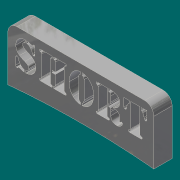
# Autodesk Inventor part: A1-19010-100-03 Tab - SHORT
Saved by Autodesk Inventor 2017 SP1 (Build 210196100, 196)
## iProperties
Created: 2014-10-23
Part Number: A1-19010-100-03 Tab - SHORT
Material: Steel, Mild
Description: 4" x 1 1/2" x 1/2" PLATE, A516 Gr.70
Document SubType Name: Modeling
Designer: Graeme_Van_Dongen
Density: 7.86 g/cm^3
Appearance: Steel
Mass: 266.205 g
Surface Area: 155.61 cm^2
Volume: 33.8683 cm^3
Author: Graeme_Van_Dongen
Autodesk Inventor part; units mm, degrees
ref_plane "YZ Plane" through (0, 0, 0) normal (1, 0, 0) x (0, 1, 0)
ref_plane "XZ Plane" through (0, 0, 0) normal (0, 1, 0) x (-1, 0, 0)
ref_plane "XY Plane" through (0, 0, 0) normal (0, 0, 1) x (1, 0, 0)
sketch "Sketch1" plane through (0, 0, 0) normal (0, 0, 1) x (1, 0, 0)
  arc A0 (50.8, 543.7321) -> (-50.8, 543.7321) centre (0, 0) ccw
  line L0 (50.8, 543.7321) -> (50.8, 581.8321)
  line L1 (50.8, 581.8321) -> (-50.8, 581.8321)
  line L2 (-50.8, 581.8321) -> (-50.8, 543.7321)
  point P0 (0, 581.8321)
  dimension "d0" = 101.6
  dimension "d1" = 38.1
  dimension "d2" = 546.1
  constraints: 6 end point, 2 parallel, 2 point on circle, 1 centre point, 1 coincident, 1 midpoint, 1 perpendicular, 1 vertical, 1 vertical alignment
  measures "d0" distance of L0.end L1.end
  measures "d1" distance of L0.start L0.end
  measures "d2" radius of A0
extrude "Extrusion1" add sketch "Sketch1" along normal mid plane 12.7
sketch "Sketch2" plane through (0, 0, 6.35) normal (0, 0, 1) x (1, 0, 0)
  line L0 (-46.29, 576.8125) -> (46.3638, 576.8125) construction
  line L1 (46.3638, 576.8125) -> (46.3638, 557.0018) construction
  line L2 (46.3638, 557.0018) -> (-46.29, 557.0018) construction
  line L3 (-46.29, 557.0018) -> (-46.29, 576.8125) construction
  line L4 (-38.7163, 576.8125) -> (-38.7163, 575.2084)
  spline S0 degree 2 poles (-38.7163, 575.2084) (-39.5762, 574.9604) (-40.4857, 573.9682) (-40.4857, 573.2571) knots 0 0 0 1 2 2 2
  spline S1 degree 2 poles (-40.4857, 573.2571) (-40.4857, 572.546) (-39.725, 571.5042) (-38.8816, 571.0247) knots 0 0 0 1 2 2 2
  spline S2 degree 2 poles (-38.8816, 571.0247) (-38.3029, 570.7105) (-36.2358, 569.801) knots 0 0 0 1 1 1
  spline S3 degree 2 poles (-36.2358, 569.801) (-34.979, 569.2553) (-33.6065, 568.3789) (-32.9781, 567.7174) knots 0 0 0 1 2 2 2
  spline S4 degree 2 poles (-32.9781, 567.7174) (-31.341, 565.9976) (-31.341, 563.5998) knots 0 0 0 1 1 1
  spline S5 degree 2 poles (-31.341, 563.5998) (-31.341, 561.8139) (-33.127, 558.8208) (-34.6814, 557.9609) knots 0 0 0 1 2 2 2
  spline S6 degree 2 poles (-34.6814, 557.9609) (-35.5247, 557.5144) (-37.5257, 557.0018) (-38.3855, 557.0018) knots 0 0 0 1 2 2 2
  line L5 (-38.3855, 557.0018) -> (-38.3855, 558.5893)
  spline S7 degree 2 poles (-38.3855, 558.5893) (-37.1784, 558.8869) (-36.1035, 559.9287) (-36.1035, 560.8217) knots 0 0 0 1 2 2 2
  spline S8 degree 2 poles (-36.1035, 560.8217) (-36.1035, 561.7643) (-36.9469, 562.4753) knots 0 0 0 1 1 1
  spline S9 degree 2 poles (-36.9469, 562.4753) (-37.4926, 562.9384) (-39.0635, 563.6164) knots 0 0 0 1 1 1
  spline S10 degree 2 poles (-39.0635, 563.6164) (-40.7668, 564.377) (-42.0401, 565.022) (-42.6354, 565.4519) knots 0 0 0 1 2 2 2
  spline S11 degree 2 poles (-42.6354, 565.4519) (-45.2482, 567.3205) (-45.2482, 570.4294) knots 0 0 0 1 1 1
  spline S12 degree 2 poles (-45.2482, 570.4294) (-45.2482, 572.0169) (-43.9418, 574.7123) (-42.7677, 575.5391) knots 0 0 0 1 2 2 2
  spline S13 degree 2 poles (-42.7677, 575.5391) (-41.1306, 576.6802) (-38.7163, 576.8125) knots 0 0 0 1 1 1
  line L6 (-39.4439, 558.5893) -> (-39.4439, 557.0018)
  spline S14 degree 2 poles (-39.4439, 557.0018) (-40.5849, 557.0018) (-41.974, 557.6467) knots 0 0 0 1 1 1
  spline S15 degree 2 poles (-41.974, 557.6467) (-42.4866, 557.8947) (-42.8835, 558.027) (-43.0654, 558.027) knots 0 0 0 1 2 2 2
  spline S16 degree 2 poles (-43.0654, 558.027) (-43.3299, 558.027) (-43.6111, 557.8451) (-43.9253, 557.4813) knots 0 0 0 1 2 2 2
  spline S17 degree 2 poles (-43.9253, 557.4813) (-44.1733, 557.1837) (-44.471, 557.1837) knots 0 0 0 1 1 1
  spline S18 degree 2 poles (-44.471, 557.1837) (-45.2482, 557.1837) (-45.2482, 558.3908) knots 0 0 0 1 1 1
  line L7 (-45.2482, 558.3908) -> (-45.2482, 563.4675)
  spline S19 degree 2 poles (-45.2482, 563.4675) (-45.2482, 563.8479) (-44.8017, 564.3936) (-44.471, 564.4101) knots 0 0 0 1 2 2 2
  spline S20 degree 2 poles (-44.471, 564.4101) (-44.1568, 564.4266) (-43.8095, 564.0463) (-43.6772, 563.5668) knots 0 0 0 1 2 2 2
  spline S21 degree 2 poles (-43.6772, 563.5668) (-43.363, 562.3761) (-42.1559, 560.276) (-41.3456, 559.5649) knots 0 0 0 1 2 2 2
  spline S22 degree 2 poles (-41.3456, 559.5649) (-40.5188, 558.8043) (-39.4439, 558.5893) knots 0 0 0 1 1 1
  line L8 (-37.6083, 575.2084) -> (-37.6083, 576.7463)
  spline S23 degree 2 poles (-37.6083, 576.7463) (-36.765, 576.6802) (-35.5413, 576.3494) (-34.4168, 575.8699) knots 0 0 0 1 2 2 2
  spline S24 degree 2 poles (-34.4168, 575.8699) (-34.1357, 575.7541) (-33.9538, 575.7541) knots 0 0 0 1 1 1
  spline S25 degree 2 poles (-33.9538, 575.7541) (-33.6892, 575.7541) (-33.5569, 575.936) knots 0 0 0 1 1 1
  line L9 (-33.5569, 575.936) -> (-33.2592, 576.3494)
  spline S26 degree 2 poles (-33.2592, 576.3494) (-33.0277, 576.6636) (-32.7135, 576.6636) knots 0 0 0 1 1 1
  spline S27 degree 2 poles (-32.7135, 576.6636) (-32.3332, 576.6636) (-31.9859, 576.1179) (-31.9859, 575.5391) knots 0 0 0 1 2 2 2
  line L10 (-31.9859, 575.5391) -> (-31.9859, 570.9255)
  spline S28 degree 2 poles (-31.9859, 570.9255) (-31.9859, 570.5121) (-32.449, 569.9994) (-32.8128, 569.9994) knots 0 0 0 1 2 2 2
  spline S29 degree 2 poles (-32.8128, 569.9994) (-33.0939, 569.9994) (-33.3254, 570.1813) knots 0 0 0 1 1 1
  spline S30 degree 2 poles (-33.3254, 570.1813) (-33.4577, 570.2971) (-33.6065, 570.6113) (-33.6727, 570.9916) knots 0 0 0 1 2 2 2
  spline S31 degree 2 poles (-33.6727, 570.9916) (-33.8215, 571.6862) (-34.5822, 573.1248) (-35.0783, 573.7036) knots 0 0 0 1 2 2 2
  spline S32 degree 2 poles (-35.0783, 573.7036) (-36.087, 574.8446) (-37.6083, 575.2084) knots 0 0 0 1 1 1
  line L11 (-20.0466, 567.8001) -> (-17.7811, 567.8001)
  line L12 (-17.7811, 567.8001) -> (-17.7811, 573.8855)
  spline S33 degree 2 poles (-17.7811, 573.8855) (-17.7811, 574.6792) (-18.178, 574.8115) knots 0 0 0 1 1 1
  line L13 (-18.178, 574.8115) -> (-18.6245, 574.9438)
  spline S34 degree 2 poles (-18.6245, 574.9438) (-19.1536, 575.1257) (-19.1536, 575.7045) knots 0 0 0 1 1 1
  spline S35 degree 2 poles (-19.1536, 575.7045) (-19.1536, 576.4321) (-18.1615, 576.4321) knots 0 0 0 1 1 1
  line L14 (-18.1615, 576.4321) -> (-17.7977, 576.4321)
  line L15 (-17.7977, 576.4321) -> (-11.5799, 576.4321)
  line L16 (-11.5799, 576.4321) -> (-11.1996, 576.4321)
  spline S36 degree 2 poles (-11.1996, 576.4321) (-10.1578, 576.4321) (-10.1578, 575.7045) knots 0 0 0 1 1 1
  spline S37 degree 2 poles (-10.1578, 575.7045) (-10.1578, 575.1257) (-10.7201, 574.9438) knots 0 0 0 1 1 1
  spline S38 degree 2 poles (-10.7201, 574.9438) (-11.1831, 574.795) (-11.3319, 574.7289) (-11.4146, 574.5966) knots 0 0 0 1 2 2 2
  spline S39 degree 2 poles (-11.4146, 574.5966) (-11.5799, 574.3816) (-11.5799, 573.8855) knots 0 0 0 1 1 1
  line L17 (-11.5799, 573.8855) -> (-11.5799, 559.9783)
  spline S40 degree 2 poles (-11.5799, 559.9783) (-11.5799, 559.2011) (-11.1665, 559.0358) knots 0 0 0 1 1 1
  line L18 (-11.1665, 559.0358) -> (-10.7201, 558.8869)
  spline S41 degree 2 poles (-10.7201, 558.8869) (-10.1578, 558.705) (-10.1578, 558.1263) knots 0 0 0 1 1 1
  spline S42 degree 2 poles (-10.1578, 558.1263) (-10.1578, 557.3821) (-11.1996, 557.3821) knots 0 0 0 1 1 1
  line L19 (-11.1996, 557.3821) -> (-11.5799, 557.3821)
  line L20 (-11.5799, 557.3821) -> (-17.7977, 557.3821)
  line L21 (-17.7977, 557.3821) -> (-18.178, 557.3821)
  spline S43 degree 2 poles (-18.178, 557.3821) (-19.1536, 557.3821) (-19.1536, 558.1263) knots 0 0 0 1 1 1
  spline S44 degree 2 poles (-19.1536, 558.1263) (-19.1536, 558.705) (-18.6245, 558.8869) knots 0 0 0 1 1 1
  line L22 (-18.6245, 558.8869) -> (-18.178, 559.0358)
  spline S45 degree 2 poles (-18.178, 559.0358) (-17.7811, 559.1681) (-17.7811, 559.9783) knots 0 0 0 1 1 1
  line L23 (-17.7811, 559.9783) -> (-17.7811, 566.411)
  line L24 (-17.7811, 566.411) -> (-20.0466, 566.411)
  line L25 (-20.0466, 566.411) -> (-20.0466, 567.8001)
  line L26 (-21.2042, 557.3821) -> (-27.4384, 557.3821)
  line L27 (-27.4384, 557.3821) -> (-27.8022, 557.3821)
  spline S46 degree 2 poles (-27.8022, 557.3821) (-28.2983, 557.3821) (-28.844, 557.7625) (-28.844, 558.1097) knots 0 0 0 1 2 2 2
  spline S47 degree 2 poles (-28.844, 558.1097) (-28.844, 558.672) (-28.2818, 558.8539) knots 0 0 0 1 1 1
  spline S48 degree 2 poles (-28.2818, 558.8539) (-27.8188, 559.0192) (-27.6699, 559.0854) (-27.5872, 559.2177) knots 0 0 0 1 2 2 2
  spline S49 degree 2 poles (-27.5872, 559.2177) (-27.4219, 559.4326) (-27.4219, 559.9287) knots 0 0 0 1 1 1
  line L28 (-27.4219, 559.9287) -> (-27.4219, 573.8855)
  spline S50 degree 2 poles (-27.4219, 573.8855) (-27.4219, 574.3816) (-27.5872, 574.5966) knots 0 0 0 1 1 1
  spline S51 degree 2 poles (-27.5872, 574.5966) (-27.6699, 574.7289) (-27.8188, 574.795) (-28.2818, 574.9438) knots 0 0 0 1 2 2 2
  spline S52 degree 2 poles (-28.2818, 574.9438) (-28.844, 575.1257) (-28.844, 575.7045) knots 0 0 0 1 1 1
  spline S53 degree 2 poles (-28.844, 575.7045) (-28.844, 576.0518) (-28.2983, 576.4321) (-27.8022, 576.4321) knots 0 0 0 1 2 2 2
  line L29 (-27.8022, 576.4321) -> (-27.4384, 576.4321)
  line L30 (-27.4384, 576.4321) -> (-21.2042, 576.4321)
  line L31 (-21.2042, 576.4321) -> (-20.8404, 576.4321)
  spline S54 degree 2 poles (-20.8404, 576.4321) (-19.8482, 576.4321) (-19.8482, 575.7045) knots 0 0 0 1 1 1
  spline S55 degree 2 poles (-19.8482, 575.7045) (-19.8482, 575.1257) (-20.3773, 574.9438) knots 0 0 0 1 1 1
  line L32 (-20.3773, 574.9438) -> (-20.8073, 574.8115)
  spline S56 degree 2 poles (-20.8073, 574.8115) (-21.2207, 574.6792) (-21.2207, 573.8855) knots 0 0 0 1 1 1
  line L33 (-21.2207, 573.8855) -> (-21.2207, 559.9287)
  spline S57 degree 2 poles (-21.2207, 559.9287) (-21.2207, 559.135) (-20.8073, 559.0027) knots 0 0 0 1 1 1
  line L34 (-20.8073, 559.0027) -> (-20.3773, 558.8539)
  spline S58 degree 2 poles (-20.3773, 558.8539) (-19.8482, 558.6885) (-19.8482, 558.1097) knots 0 0 0 1 1 1
  spline S59 degree 2 poles (-19.8482, 558.1097) (-19.8482, 557.3821) (-20.8404, 557.3821) knots 0 0 0 1 1 1
  line L35 (-20.8404, 557.3821) -> (-21.2042, 557.3821)
  line L36 (0.9216, 575.3076) -> (0.9216, 576.8125)
  spline S60 degree 2 poles (0.9216, 576.8125) (2.4264, 576.7463) (4.9234, 575.6549) (5.9983, 574.5966) knots 0 0 0 1 2 2 2
  spline S61 degree 2 poles (5.9983, 574.5966) (8.8426, 571.8184) (8.8426, 566.8906) knots 0 0 0 1 1 1
  spline S62 degree 2 poles (8.8426, 566.8906) (8.8426, 562.0454) (6.1306, 559.3334) knots 0 0 0 1 1 1
  spline S63 degree 2 poles (6.1306, 559.3334) (4.0305, 557.2498) (0.9216, 557.0018) knots 0 0 0 1 1 1
  line L37 (0.9216, 557.0018) -> (0.9216, 558.5397)
  spline S64 degree 2 poles (0.9216, 558.5397) (1.2854, 558.6223) (1.6823, 558.8869) (1.8477, 559.135) knots 0 0 0 1 2 2 2
  spline S65 degree 2 poles (1.8477, 559.135) (2.228, 559.7138) (2.228, 560.8713) knots 0 0 0 1 1 1
  line L38 (2.228, 560.8713) -> (2.228, 573.3398)
  spline S66 degree 2 poles (2.228, 573.3398) (2.228, 574.0839) (1.9799, 574.5139) knots 0 0 0 1 1 1
  spline S67 degree 2 poles (1.9799, 574.5139) (1.8146, 574.8115) (1.3516, 575.1423) (0.9216, 575.3076) knots 0 0 0 1 2 2 2
  spline S68 degree 2 poles (-0.2194, 575.3076) (-0.9305, 575.0431) (-1.5092, 574.1832) (-1.5092, 573.3398) knots 0 0 0 1 2 2 2
  line L39 (-1.5092, 573.3398) -> (-1.5092, 560.8713)
  spline S69 degree 2 poles (-1.5092, 560.8713) (-1.5092, 559.6476) (-1.1785, 559.135) knots 0 0 0 1 1 1
  spline S70 degree 2 poles (-1.1785, 559.135) (-0.9139, 558.7216) (-0.2194, 558.5397) knots 0 0 0 1 1 1
  line L40 (-0.2194, 558.5397) -> (-0.2194, 557.0018)
  spline S71 degree 2 poles (-0.2194, 557.0018) (-3.3117, 557.2498) (-5.4118, 559.3334) knots 0 0 0 1 1 1
  spline S72 degree 2 poles (-5.4118, 559.3334) (-8.1238, 562.0454) (-8.1238, 566.8906) knots 0 0 0 1 1 1
  spline S73 degree 2 poles (-8.1238, 566.8906) (-8.1238, 569.3214) (-6.6852, 573.2406) (-5.2796, 574.5966) knots 0 0 0 1 2 2 2
  spline S74 degree 2 poles (-5.2796, 574.5966) (-4.2047, 575.6549) (-1.7242, 576.7463) (-0.2194, 576.8125) knots 0 0 0 1 2 2 2
  line L41 (-0.2194, 576.8125) -> (-0.2194, 575.3076)
  line L42 (18.1857, 576.4321) -> (18.1857, 560.0279)
  spline S75 degree 2 poles (18.1857, 560.0279) (18.1857, 559.4822) (18.4006, 559.2507) knots 0 0 0 1 1 1
  spline S76 degree 2 poles (18.4006, 559.2507) (18.4999, 559.1184) (18.6983, 559.0358) (19.244, 558.9035) knots 0 0 0 1 2 2 2
  spline S77 degree 2 poles (19.244, 558.9035) (19.922, 558.7546) (19.922, 558.1428) knots 0 0 0 1 1 1
  spline S78 degree 2 poles (19.922, 558.1428) (19.922, 557.779) (19.5582, 557.5475) knots 0 0 0 1 1 1
  spline S79 degree 2 poles (19.5582, 557.5475) (19.2936, 557.3821) (18.6818, 557.3821) knots 0 0 0 1 1 1
  line L43 (18.6818, 557.3821) -> (18.2022, 557.3821)
  line L44 (18.2022, 557.3821) -> (11.968, 557.3821)
  line L45 (11.968, 557.3821) -> (11.6042, 557.3821)
  spline S80 degree 2 poles (11.6042, 557.3821) (11.1081, 557.3821) (10.5624, 557.7625) (10.5624, 558.1097) knots 0 0 0 1 2 2 2
  spline S81 degree 2 poles (10.5624, 558.1097) (10.5624, 558.672) (11.1246, 558.8539) knots 0 0 0 1 1 1
  spline S82 degree 2 poles (11.1246, 558.8539) (11.5876, 559.0192) (11.7365, 559.0854) (11.8191, 559.2177) knots 0 0 0 1 2 2 2
  spline S83 degree 2 poles (11.8191, 559.2177) (11.9845, 559.4326) (11.9845, 559.9287) knots 0 0 0 1 1 1
  line L46 (11.9845, 559.9287) -> (11.9845, 573.8855)
  spline S84 degree 2 poles (11.9845, 573.8855) (11.9845, 574.3816) (11.8191, 574.5966) knots 0 0 0 1 1 1
  spline S85 degree 2 poles (11.8191, 574.5966) (11.7365, 574.7289) (11.5876, 574.795) (11.1246, 574.9438) knots 0 0 0 1 2 2 2
  spline S86 degree 2 poles (11.1246, 574.9438) (10.5624, 575.1257) (10.5624, 575.7045) knots 0 0 0 1 1 1
  spline S87 degree 2 poles (10.5624, 575.7045) (10.5624, 576.0518) (11.1081, 576.4321) (11.6042, 576.4321) knots 0 0 0 1 2 2 2
  line L47 (11.6042, 576.4321) -> (11.968, 576.4321)
  line L48 (11.968, 576.4321) -> (18.1857, 576.4321)
  spline S88 degree 2 poles (22.4686, 566.7087) (23.7419, 566.5268) (25.131, 566.0472) (25.6932, 565.6338) knots 0 0 0 1 2 2 2
  spline S89 degree 2 poles (25.6932, 565.6338) (26.272, 565.2039) (26.9004, 564.0132) (26.9004, 563.3352) knots 0 0 0 1 2 2 2
  line L49 (26.9004, 563.3352) -> (26.9004, 560.4579)
  spline S90 degree 2 poles (26.9004, 560.4579) (26.9004, 559.9949) (27.198, 559.9949) knots 0 0 0 1 1 1
  spline S91 degree 2 poles (27.198, 559.9949) (27.2973, 559.9949) (27.4626, 560.1272) (27.5949, 560.3091) knots 0 0 0 1 2 2 2
  spline S92 degree 2 poles (27.5949, 560.3091) (27.9422, 560.7886) (28.306, 560.7886) knots 0 0 0 1 1 1
  spline S93 degree 2 poles (28.306, 560.7886) (28.5375, 560.7886) (29.0171, 560.2925) (29.0171, 560.0279) knots 0 0 0 1 2 2 2
  spline S94 degree 2 poles (29.0171, 560.0279) (29.0171, 559.598) (28.1902, 558.3578) (27.5784, 557.8617) knots 0 0 0 1 2 2 2
  spline S95 degree 2 poles (27.5784, 557.8617) (27.0161, 557.4152) (25.6767, 557.0018) (24.7672, 557.0018) knots 0 0 0 1 2 2 2
  spline S96 degree 2 poles (24.7672, 557.0018) (22.9316, 557.0018) (20.8646, 559.1184) (20.8646, 560.9871) knots 0 0 0 1 2 2 2
  line L50 (20.8646, 560.9871) -> (20.8646, 563.3352)
  spline S97 degree 2 poles (20.8646, 563.3352) (20.8646, 564.1125) (20.848, 564.2447) knots 0 0 0 1 1 1
  spline S98 degree 2 poles (20.848, 564.2447) (20.7819, 564.807) (20.4512, 565.2039) knots 0 0 0 1 1 1
  spline S99 degree 2 poles (20.4512, 565.2039) (20.0543, 565.7) (19.2936, 565.7826) knots 0 0 0 1 1 1
  line L51 (19.2936, 565.7826) -> (19.2936, 567.2709)
  spline S100 degree 2 poles (19.2936, 567.2709) (20.0543, 567.3867) (20.3685, 567.6678) knots 0 0 0 1 1 1
  spline S101 degree 2 poles (20.3685, 567.6678) (20.6496, 567.9158) (20.8646, 568.5608) (20.8646, 569.1891) knots 0 0 0 1 2 2 2
  line L52 (20.8646, 569.1891) -> (20.8646, 572.8933)
  spline S102 degree 2 poles (20.8646, 572.8933) (20.8646, 573.7697) (20.1866, 574.6296) (19.2936, 574.8777) knots 0 0 0 1 2 2 2
  line L53 (19.2936, 574.8777) -> (19.2936, 576.4321)
  line L54 (19.2936, 576.4321) -> (19.6574, 576.4321)
  spline S103 degree 2 poles (19.6574, 576.4321) (21.1953, 576.4321) (22.2867, 576.3164) knots 0 0 0 1 1 1
  spline S104 degree 2 poles (22.2867, 576.3164) (23.9073, 576.1675) (25.1806, 575.258) knots 0 0 0 1 1 1
  spline S105 degree 2 poles (25.1806, 575.258) (26.9996, 573.9682) (26.9996, 571.5539) knots 0 0 0 1 1 1
  spline S106 degree 2 poles (26.9996, 571.5539) (26.9996, 569.586) (25.7759, 568.3292) knots 0 0 0 1 1 1
  spline S107 degree 2 poles (25.7759, 568.3292) (25.2633, 567.8001) (23.8742, 567.1386) (22.4686, 566.7087) knots 0 0 0 1 2 2 2
  line L55 (40.9729, 576.4321) -> (40.9729, 560.0279)
  spline S108 degree 2 poles (40.9729, 560.0279) (40.9729, 559.4822) (41.1879, 559.2507) knots 0 0 0 1 1 1
  spline S109 degree 2 poles (41.1879, 559.2507) (41.2871, 559.1184) (41.4855, 559.0358) (42.0312, 558.9035) knots 0 0 0 1 2 2 2
  spline S110 degree 2 poles (42.0312, 558.9035) (42.7092, 558.7546) (42.7092, 558.1428) knots 0 0 0 1 1 1
  spline S111 degree 2 poles (42.7092, 558.1428) (42.7092, 557.779) (42.3454, 557.5475) knots 0 0 0 1 1 1
  spline S112 degree 2 poles (42.3454, 557.5475) (42.0809, 557.3821) (41.4525, 557.3821) knots 0 0 0 1 1 1
  line L56 (41.4525, 557.3821) -> (40.9895, 557.3821)
  line L57 (40.9895, 557.3821) -> (34.7552, 557.3821)
  line L58 (34.7552, 557.3821) -> (34.2922, 557.3821)
  spline S113 degree 2 poles (34.2922, 557.3821) (33.6803, 557.3821) (33.052, 557.7625) (33.052, 558.1428) knots 0 0 0 1 2 2 2
  spline S114 degree 2 poles (33.052, 558.1428) (33.052, 558.7546) (33.7299, 558.9035) knots 0 0 0 1 1 1
  spline S115 degree 2 poles (33.7299, 558.9035) (34.2756, 559.0358) (34.4576, 559.1184) (34.5568, 559.2507) knots 0 0 0 1 2 2 2
  spline S116 degree 2 poles (34.5568, 559.2507) (34.7717, 559.4822) (34.7717, 560.0279) knots 0 0 0 1 1 1
  line L59 (34.7717, 560.0279) -> (34.7717, 576.4321)
  line L60 (34.7717, 576.4321) -> (40.9729, 576.4321)
  line L61 (45.785, 576.4321) -> (45.785, 570.727)
  spline S117 degree 2 poles (45.785, 570.727) (45.785, 570.3136) (45.322, 569.8175) (44.9582, 569.8175) knots 0 0 0 1 2 2 2
  spline S118 degree 2 poles (44.9582, 569.8175) (44.6109, 569.8175) (44.1479, 570.2806) (44.0818, 570.6774) knots 0 0 0 1 2 2 2
  line L62 (44.0818, 570.6774) -> (43.9495, 571.5373)
  spline S119 degree 2 poles (43.9495, 571.5373) (43.7345, 572.8272) (43.1392, 573.7863) knots 0 0 0 1 1 1
  spline S120 degree 2 poles (43.1392, 573.7863) (42.7589, 574.3651) (42.1139, 574.7454) knots 0 0 0 1 1 1
  line L63 (42.1139, 574.7454) -> (42.1139, 576.4321)
  line L64 (42.1139, 576.4321) -> (45.785, 576.4321)
  line L65 (29.9762, 576.4321) -> (33.6473, 576.4321)
  line L66 (33.6473, 576.4321) -> (33.6473, 574.7454)
  spline S121 degree 2 poles (33.6473, 574.7454) (32.9858, 574.3651) (32.622, 573.7863) knots 0 0 0 1 1 1
  spline S122 degree 2 poles (32.622, 573.7863) (32.0267, 572.8272) (31.8117, 571.5373) knots 0 0 0 1 1 1
  line L67 (31.8117, 571.5373) -> (31.6794, 570.6774)
  spline S123 degree 2 poles (31.6794, 570.6774) (31.6133, 570.2806) (31.1503, 569.8175) (30.803, 569.8175) knots 0 0 0 1 2 2 2
  spline S124 degree 2 poles (30.803, 569.8175) (30.4392, 569.8175) (29.9762, 570.3136) (29.9762, 570.727) knots 0 0 0 1 2 2 2
  line L68 (29.9762, 570.727) -> (29.9762, 576.4321)
  point P0 (0, 0)
  constraints: 2 other
extrude "Extrusion2" cut sketch "Sketch2" against normal through all
fillet "Fillet1" radius 6.35 2 edges at (-50.8, 581.8321, 0) (50.8, 581.8321, 0)
body "Solid1"
